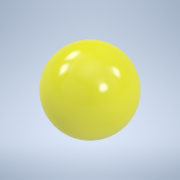
# Autodesk Inventor part: Ball
Saved by Autodesk Inventor 2020 (Build 240168000, 168)
## iProperties
Created: 2020-01-19
Part Number: Ball
Material: Generic
Document SubType Name: Modeling
Designer: srini
Density: 1 g/cm^3
Appearance: Yellow
Author: srini
Autodesk Inventor part; units mm, degrees
ref_plane "YZ Plane" through (0, 0, 0) normal (1, 0, 0) x (0, 1, 0)
ref_plane "XZ Plane" through (0, 0, 0) normal (0, 1, 0) x (-1, 0, 0)
ref_plane "XY Plane" through (0, 0, 0) normal (0, 0, 1) x (1, 0, 0)
sketch "Sketch1" plane through (0, 0, 0) normal (0, 0, 1) x (1, 0, 0)
  arc A0 (0, -88.9) -> (0, 88.9) centre (0, 0) ccw
  line L0 (0, 88.9) -> (0, -88.9)
  arc A1 (0, 88.9) -> (0, -88.9) centre (0, 0) ccw
  dimension "d0" = 177.8
  constraints: 4 point on circle, 2 centre point, 2 end point, 1 coincident, 1 midpoint, 1 vertical
  measures "d0" diameter of A0
revolve "Revolution1" add sketch "Sketch1" angle 360 about axis through (0, 88.9, 0) along (0, -1, 0) contours L0 A0
body "Solid1"
